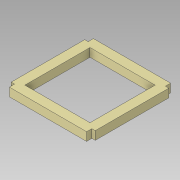
# Autodesk Inventor part: Carriage Sheet
Saved by Autodesk Inventor 2016 (Build 200138000, 138)
## iProperties
Created: 2017-05-17
Part Number: Carriage Sheet
Material: Generic
Document SubType Name: Modeling
Designer: 31745
Density: 1 g/cm^3
Appearance: Default
Author: 31745
Autodesk Inventor part; units mm, degrees
ref_plane "YZ Plane" through (0, 0, 0) normal (1, 0, 0) x (0, 1, 0)
ref_plane "XZ Plane" through (0, 0, 0) normal (0, 1, 0) x (-1, 0, 0)
ref_plane "XY Plane" through (0, 0, 0) normal (0, 0, 1) x (1, 0, 0)
sketch "Sketch1" plane through (0, 0, 0) normal (0, 1, 0) x (-1, 0, 0)
  line L0 (0, 0) -> (-254, 0)
  line L1 (-254, 0) -> (-254, -254)
  line L2 (-254, -254) -> (0, -254)
  line L3 (0, -254) -> (0, 0)
  line L4 (0, -15.875) -> (-10.287, -15.875)
  line L5 (-10.287, -15.875) -> (-10.287, 0)
  line L6 (-243.713, 0) -> (-243.713, -15.875)
  line L7 (-243.713, -15.875) -> (-254, -15.875)
  line L8 (-243.713, -254) -> (-243.713, -238.125)
  line L9 (-243.713, -238.125) -> (-254, -238.125)
  line L10 (-10.287, -254) -> (-10.287, -238.125)
  line L11 (-10.287, -238.125) -> (0, -238.125)
  dimension "d0" = 254
  dimension "d1" = 254
  dimension "d13" = 10.287
  dimension "d14" = 10.287
  dimension "d15" = 15.875
  dimension "d16" = 15.875
  constraints: 24 end point, 12 point on line, 5 perpendicular, 2 horizontal, 2 horizontal alignment, 2 parallel, 1 vertical, 1 vertical alignment
  measures "d0" distance of L2.end L1.end
  measures "d1" distance of L1.end L0.end
  measures "d13" distance of L10.end L11.end
  measures "d14" distance of L8.end L9.end
  measures "d15" distance of L8.start L8.end
  measures "d16" distance of L4.end L5.end
extrude "Extrusion1" add sketch "Sketch1" along normal blind 25.4 contours L5 L4 L3 L11 L10 L2 L8 L9 L1 L7 L6 L0
sketch "Sketch2" plane through (0, 25.4, 0) normal (0, 1, 0) x (1, 0, 0)
  line L0 (28.575, 28.575) -> (225.425, 28.575)
  line L1 (225.425, 28.575) -> (225.425, 225.425)
  line L2 (225.425, 225.425) -> (28.575, 225.425)
  line L3 (28.575, 225.425) -> (28.575, 28.575)
  line L4 (0, 15.875) -> (10.287, 15.875) projected
  line L5 (10.287, 15.875) -> (10.287, 0) projected
  line L6 (10.287, 0) -> (243.713, 0) projected
  line L7 (243.713, 0) -> (243.713, 15.875) projected
  line L8 (243.713, 15.875) -> (254, 15.875) projected
  line L9 (254, 15.875) -> (254, 238.125) projected
  line L10 (254, 238.125) -> (243.713, 238.125) projected
  line L11 (243.713, 238.125) -> (243.713, 254) projected
  line L12 (243.713, 254) -> (10.287, 254) projected
  line L13 (10.287, 254) -> (10.287, 238.125) projected
  line L14 (10.287, 238.125) -> (0, 238.125) projected
  line L15 (0, 238.125) -> (0, 15.875) projected
  point P0 (0, 0)
  point P1 (127, 28.575)
  point P2 (127, 0)
  point P3 (28.575, 127)
  point P4 (0, 127)
  dimension "d9" = 196.85
  dimension "d10" = 196.85
  constraints: 8 end point, 4 midpoint, 2 parallel, 1 horizontal, 1 horizontal alignment, 1 perpendicular, 1 vertical alignment
  measures "d9" distance of L2.end L0.start
  measures "d10" distance of L1.end L2.end
extrude "Extrusion2" cut sketch "Sketch2" against normal through all contours L3 L2 L1 L0
fillet "Fillet1" radius 6.35 1 edges at (10.287, 12.7, 0)
sketch "Sketch3" plane through (0, 25.4, 0) normal (0, 1, 0) x (1, 0, 0)
  circle A0 centre (50.8, 9.525) radius 7.5 projected
  circle A1 centre (50.8, 244.475) radius 7.5 projected
  circle A2 centre (203.2, 244.475) radius 4 projected
  circle A3 centre (203.2, 244.475) radius 7.5 projected
  circle A4 centre (203.2, 9.525) radius 7.5 projected
  point P0 (0, 0)
hole "Hole1" at (50.8, 25.4, -9.525) at (50.8, 25.4, -244.475) at (203.2, 25.4, -9.525) at (203.2, 25.4, -244.475) direction (0, -1, 0) diameter 15 end through all
equation "\"d14\" = d13"
equation "\"d9\" = d10"
body "Solid1"
